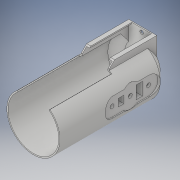
# Autodesk Inventor part: fakebattery
Saved by Autodesk Inventor 2018.3 (Build 223284000, 284)
## iProperties
Created: 2019-09-05
Part Number: fakebattery
Material: Generic
Document SubType Name: Modeling
Designer: Srinity
Density: 1 g/cm^3
Appearance: Default
Author: Srinity
Autodesk Inventor part; units mm, degrees
ref_plane "YZ Plane" through (0, 0, 0) normal (1, 0, 0) x (0, 1, 0)
sketch "Sketch1" plane through (0, 0, 0) normal (0, 0, 1) x (1, 0, 0)
  circle A0 centre (0, 0) radius 37
  line L0 (-19.52, 40.52) -> (19.52, 40.52)
  line L1 (19.52, 40.52) -> (19.52, 0)
  line L2 (19.52, 0) -> (-19.52, 0)
  line L3 (-19.52, 0) -> (-19.52, 40.52)
  dimension "d0" = 74
  dimension "d1" = 39.04
  dimension "d2" = 40.52
  constraints: 8 end point, 2 coincident, 2 parallel, 1 centre point, 1 horizontal, 1 midpoint, 1 perpendicular
  measures "d0" diameter of A0
  measures "d1" distance of L0.start L0.end
  measures "d2" distance between parallel lines of L2 L0
extrude "Extrusion1" add sketch "Sketch1" along normal blind 152.4
chamfer "Chamfer1" distance 12.7 angle 45 1 edges at (0, -37, 0)
shell "Shell1" thickness 1.67 removed faces 1 at (5.3335, -8.3183, 152.4)
sketch "Sketch2" plane through (0, 0, 152.4) normal (0, 0, 1) x (1, 0, 0)
  line L0 (-37.3244, 40.52) -> (36.3431, 40.52)
  line L1 (36.3431, 40.52) -> (36.3431, 29)
  line L2 (36.3431, 29) -> (-37.3244, 29)
  line L3 (-37.3244, 29) -> (-37.3244, 40.52)
  line L4 (-19.52, 40.52) -> (-19.52, 31.432) projected
  line L5 (19.52, 40.52) -> (-19.52, 40.52) projected
  line L6 (19.52, 31.432) -> (19.52, 40.52) projected
  point P0 (0, 0)
  dimension "d5" = 29
  constraints: 8 end point, 2 parallel, 1 collinear, 1 horizontal, 1 perpendicular
  measures "d5" distance from line of L2 point (0, 0)
extrude "Extrusion2" cut sketch "Sketch2" against normal blind 86
sketch "Sketch3" plane through (0, 0, 152.4) normal (0, 0, 1) x (1, 0, 0)
  line L0 (-13.75, 69.2366) -> (13.75, 69.2366)
  line L1 (13.75, 69.2366) -> (13.75, 23.255)
  line L2 (13.75, 23.255) -> (-13.75, 23.255)
  line L3 (-13.75, 23.255) -> (-13.75, 69.2366)
  point P0 (0, 0)
  point P1 (0, 23.255)
  dimension "d12" = 27.5
  constraints: 8 end point, 2 parallel, 1 horizontal, 1 midpoint, 1 perpendicular, 1 vertical alignment
  measures "d12" distance between parallel lines of L1 L3
extrude "Extrusion3" cut sketch "Sketch3" against normal blind 150.73
sketch "Sketch4" plane through (0, 0, 0) normal (0, 0, -1) x (-1, 0, 0)
  circle A0 centre (0, 35.52) radius 2.5
  line L0 (19.52, 40.52) -> (-19.52, 40.52) projected
  point P0 (0, 0)
  dimension "d15" = 5
  dimension "d16" = 5
  constraints: 1 centre point, 1 vertical alignment
  measures "d15" distance from line of A0.centre L0
  measures "d16" diameter of A0
extrude "Extrusion4" cut sketch "Sketch4" against normal blind 86
fillet "Fillet1" radius 0.835 2 edges at (20.1794, 29, 109.4) (-20.1794, 29, 109.4)
chamfer "Chamfer2" distance 3.175 angle 45 2 edges at (13.75, 39.685, 66.4) (-13.75, 39.685, 66.4)
chamfer "Chamfer3" distance 7.62 angle 45 2 edges at (-18.2225, 40.52, 66.4) (18.2225, 40.52, 66.4)
ref_plane "Work Plane1" through (0, 0, 93.11) normal (0, 0, 1) x (1, 0, 0)
sketch "Sketch5" plane through (0, 0, 93.11) normal (0, 0, 1) x (1, 0, 0)
  arc A0 (-22.1619, 27.5147) -> (22.1619, 27.5147) centre (0, 0) ccw projected
  line L0 (24.3, -25.646) -> (24.3, 25.646)
  arc A1 (-19.52, 14.4727) -> (19.52, 14.4727) centre (0, 0) ccw projected
  arc A2 (24.3, -25.646) -> (24.3, 25.646) centre (0, 0) ccw
  constraints: 4 point on circle, 2 end point, 1 centre point, 1 concentric, 1 tangent, 1 vertical
extrude "Extrusion5" add sketch "Sketch5" against normal up to next
ref_plane "Work Plane2" through (49.7, -25.646, 93.11) normal (-1, 0, 0) x (0, 1, 0)
sketch "Sketch6" plane through (49.7, -25.646, 93.11) normal (-1, 0, 0) x (0, 1, 0)
  line L0 (34.536, 50.565) -> (16.756, 50.565)
  line L1 (16.756, 50.565) -> (16.756, 59.455)
  line L2 (16.756, 59.455) -> (34.536, 59.455)
  line L3 (34.536, 59.455) -> (34.536, 50.565)
  circle A0 centre (25.646, 67.71) radius 2.75
  line L4 (30.726, 25.8) -> (20.566, 25.8)
  line L5 (20.566, 25.8) -> (20.566, 33.42)
  line L6 (20.566, 33.42) -> (30.726, 33.42)
  line L7 (30.726, 33.42) -> (30.726, 25.8)
  circle A1 centre (25.646, 42.31) radius 2.75
  line L8 (16.756, 55.01) -> (34.536, 55.01) construction
  line L9 (20.566, 29.61) -> (30.726, 29.61) construction
  circle A2 centre (25.646, 16.91) radius 2.75
  line L10 (1.346, 93.11) -> (40.1188, 93.11) projected
  line L11 (56.1352, 79.7183) -> (-9.684, 79.7183) projected
  line L12 (25.646, 129.8596) -> (25.646, -90.8149) projected
  point P0 (25.646, 33.42)
  point P1 (25.646, 59.455)
  point P2 (0, 79.7183)
  dimension "d30" = 8.89
  dimension "d31" = 17.78
  dimension "d33" = 5.5
  dimension "d37" = 10.16
  dimension "d38" = 7.62
  dimension "d42" = 25.4
  dimension "d53" = 12.7
  dimension "d54" = 25.4
  dimension "d56" = 25.4
  constraints: 20 end point, 6 midpoint, 4 parallel, 3 centre point, 2 horizontal, 2 perpendicular, 2 point on line, 1 vertical, 1 vertical alignment, 4 other
  measures "d30" distance of L2.end L0.start
  measures "d31" distance of L0.start L0.end
  measures "d33" diameter of A0
  measures "d37" distance of L4.start L4.end
  measures "d38" distance of L6.end L4.start
  measures "d42" distance of A0.centre A1.centre
  measures "d53" distance from line of L8 A0.centre
  measures "d54" distance between parallel lines of L8 L9
  measures "d56" distance from line of A0.centre L10
extrude "Extrusion6" cut sketch "Sketch6" along normal blind 30.48
sketch "Sketch7" plane through (49.7, -25.646, 93.11) normal (-1, 0, 0) x (0, 1, 0)
  circle A0 centre (25.646, 67.71) radius 2.75 projected
  line L0 (25.646, 16.91) -> (25.646, 67.71) construction
  line L1 (12.446, 16.91) -> (12.446, 67.71)
  line L2 (38.846, 67.71) -> (38.846, 16.91)
  arc A1 (12.446, 16.91) -> (38.846, 16.91) centre (25.646, 16.91) ccw
  arc A2 (38.846, 67.71) -> (12.446, 67.71) centre (25.646, 67.71) ccw
  circle A3 centre (25.646, 16.91) radius 2.75 projected
  circle A4 centre (25.646, 16.91) radius 2.75
  circle A5 centre (25.646, 42.31) radius 16.125
  point P0 (25.646, 93.11)
  dimension "d47" = 13.2
  dimension "d55" = 32.25
  constraints: 8 end point, 4 centre point, 4 point on circle, 4 tangent, 3 coincident, 1 concentric, 1 midpoint, 1 parallel, 1 vertical
  measures "d47" radius of A2
  measures "d55" diameter of A5
extrude "Extrusion7" cut sketch "Sketch7" along normal blind 16.51 contours A0 | L1 A5 L2 A1 | A5 L1 | L1 A5 L2 | L1 A2 L2 A5 | L2 A5 | A3
sketch "Sketch8" plane through (24.3, -25.646, 93.11) normal (-1, 0, 0) x (0, 1, 0)
  circle A0 centre (25.646, 67.71) radius 2.75 projected
  line L0 (30.2648, 67.71) -> (27.9554, 63.71)
  line L1 (27.9554, 63.71) -> (23.3366, 63.71)
  line L2 (23.3366, 63.71) -> (21.0272, 67.71)
  line L3 (21.0272, 67.71) -> (23.3366, 71.71)
  line L4 (23.3366, 71.71) -> (27.9554, 71.71)
  line L5 (27.9554, 71.71) -> (30.2648, 67.71)
  circle A1 centre (25.646, 42.31) radius 2.75 projected
  line L6 (30.2648, 42.31) -> (27.9554, 38.31)
  line L7 (27.9554, 38.31) -> (23.3366, 38.31)
  line L8 (23.3366, 38.31) -> (21.0272, 42.31)
  line L9 (21.0272, 42.31) -> (23.3366, 46.31)
  line L10 (23.3366, 46.31) -> (27.9554, 46.31)
  line L11 (27.9554, 46.31) -> (30.2648, 42.31)
  point P0 (25.646, 93.11)
  dimension "d50" = 8
  constraints: 24 end point, 2 coincident, 2 horizontal, 1 parallel, 26 other
  measures "d50" distance between parallel lines of L2 L5
extrude "Extrusion8" cut sketch "Sketch8" against normal blind 6 contours A0 | L0 L1 L2 L3 L4 L5 | A1 | L6 L7 L8 L9 L10 L11
body "Solid1"
